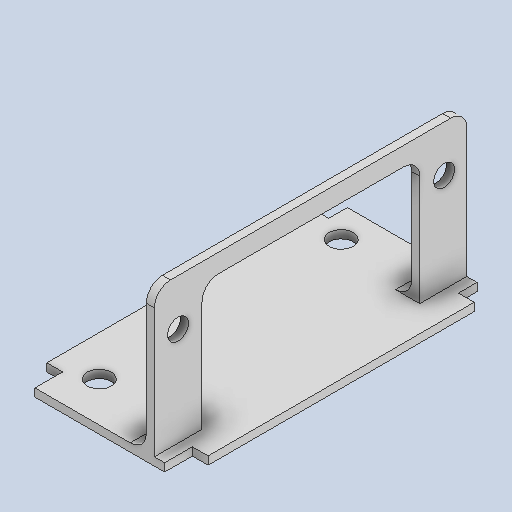
# Autodesk Inventor part: spekaer cover
Saved by Autodesk Inventor 2022.2 (Build 262287000, 287)
## iProperties
Created: 2022-02-22
Part Number: spekaer cover
Material: Generic
Document SubType Name: Modeling
Designer: ONG
Density: 1 g/cm^3
Appearance: Default
Author: ONG
Autodesk Inventor part; units mm, degrees
ref_plane "YZ Plane" through (0, 0, 0) normal (1, 0, 0) x (0, 1, 0)
ref_plane "XZ Plane" through (0, 0, 0) normal (0, 1, 0) x (-1, 0, 0)
ref_plane "XY Plane" through (0, 0, 0) normal (0, 0, 1) x (1, 0, 0)
sketch "Sketch1" plane through (0, 0, 0) normal (0, 1, 0) x (-1, 0, 0)
  line L0 (-10, -16.5) -> (10, -16.5)
  line L1 (10, -16.5) -> (10, 16.5)
  line L2 (10, 16.5) -> (-10, 16.5)
  line L3 (-10, 16.5) -> (-10, -16.5)
  line L4 (-10, -16.5) -> (10, 16.5) construction
  line L5 (10, -16.5) -> (-10, 16.5) construction
  point P0 (0, 0)
  dimension "d0" = 20
  dimension "d1" = 33
  constraints: 12 end point, 2 midpoint, 2 parallel, 1 horizontal, 1 perpendicular
  measures "d0" distance of L2.end L1.end
  measures "d1" distance of L1.end L0.end
extrude "Extrusion1" add sketch "Sketch1" along normal blind 1
sketch "Sketch2" plane through (0, 1, 0) normal (0, 1, 0) x (1, 0, 0)
  line L0 (0, 0) -> (0, 15)
  line L1 (0, 0) -> (0, -16.9855)
  line L2 (-8.0399, 11.188) -> (8.0399, 11.188)
  line L3 (8.0399, 11.188) -> (8.0399, 18.812)
  line L4 (8.0399, 18.812) -> (-8.0399, 18.812)
  line L5 (-8.0399, 18.812) -> (-8.0399, 11.188)
  line L6 (-8.0399, 11.188) -> (8.0399, 18.812) construction
  line L7 (8.0399, 11.188) -> (-8.0399, 18.812) construction
  line L8 (-8.0399, -19.9319) -> (8.0399, -19.9319)
  line L9 (8.0399, -19.9319) -> (8.0399, -14.0391)
  line L10 (8.0399, -14.0391) -> (-8.0399, -14.0391)
  line L11 (-8.0399, -14.0391) -> (-8.0399, -19.9319)
  line L12 (-8.0399, -19.9319) -> (8.0399, -14.0391) construction
  line L13 (8.0399, -19.9319) -> (-8.0399, -14.0391) construction
  dimension "d4" = 15
  constraints: 28 end point, 4 midpoint, 4 parallel, 2 horizontal, 2 perpendicular, 2 vertical, 1 point on line
  measures "d4" distance of L0.start L0.end
extrude "Extrusion2" add sketch "Sketch2" against normal blind 1
sketch "Sketch3" plane through (0, 1, 0) normal (0, 1, 0) x (1, 0, 0)
  line L0 (-8.0399, 18.812) -> (8.0399, 18.812) projected
  line L1 (6.7702, 18.812) -> (5.7702, 18.812)
  line L2 (5.7702, 18.812) -> (5.7702, 12.9733)
  line L3 (5.7702, 12.9733) -> (6.7702, 12.9733)
  line L4 (6.7702, 12.9733) -> (6.7702, 18.812)
  line L5 (8.0399, -19.9319) -> (-8.0399, -19.9319) projected
  line L6 (6.7702, -14.028) -> (5.7702, -14.028)
  line L7 (5.7702, -14.028) -> (5.7702, -19.9319)
  line L8 (5.7702, -19.9319) -> (6.7702, -19.9319)
  line L9 (6.7702, -19.9319) -> (6.7702, -14.028)
  point P0 (0, 0)
  dimension "d7" = 1
  constraints: 16 end point, 4 parallel, 2 horizontal, 2 perpendicular, 2 point on line
  measures "d7" distance of L3.end L2.end
extrude "Extrusion3" add sketch "Sketch3" along normal blind 18
fillet "Fillet1" radius 2 2 edges at (5.7702, 1, -15.8927) (5.7702, 1, 16.9799)
sketch "Sketch4" plane through (6.7702, 1, -12.9733) normal (1, 0, 0) x (0, 0, -1)
  circle A0 centre (2.9948, 12.1931) radius 1.1455
  circle A1 centre (-29.9076, 12.1931) radius 1.1628
  point P0 (-12.9733, -1)
  constraints: 2 centre point
extrude "Extrusion4" cut sketch "Sketch4" against normal blind 15
sketch "Sketch5" plane through (6.7702, 19, 14.028) normal (0, 0, -1) x (-1, 0, 0)
  line L0 (1, -16) -> (1, 0) projected
  line L1 (0, 0) -> (1, 0)
  line L2 (1, 0) -> (1, -2.3095)
  line L3 (1, -2.3095) -> (0, -2.3095)
  line L4 (0, -2.3095) -> (0, 0)
  point P0 (6.7702, -19)
  constraints: 8 end point, 2 parallel, 1 horizontal, 1 perpendicular, 1 point on line
extrude "Extrusion5" add sketch "Sketch5" along normal blind 30
fillet "Fillet2" radius 2 4 edges at (6.2702, 19, -18.812) (6.2702, 19, 19.9319) (6.2702, 16.6905, 14.028) (6.2702, 16.6905, -12.9733)
sketch "Sketch7" plane through (0, 1, 0) normal (0, 1, 0) x (1, 0, 0)
  line L0 (0, 0) -> (-5.0872, 0)
  line L1 (0, 0) -> (-5, 0)
  line L2 (-5, 0) -> (-5, -15)
  line L3 (-5, -15) -> (-5, 15)
  circle A0 centre (-5, 15) radius 1.5
  circle A1 centre (-5, -15) radius 1.5
  dimension "d19" = 5
  dimension "d20" = 15
  dimension "d21" = 30
  dimension "d22" = 3
  dimension "d23" = 3
  constraints: 8 end point, 2 centre point, 2 coincident, 2 point on line, 1 horizontal, 1 perpendicular
  measures "d19" distance of L0.start L1.end
  measures "d20" distance of L1.end L2.end
  measures "d21" distance of L2.end L3.end
  measures "d22" diameter of A0
  measures "d23" diameter of A1
extrude "Extrusion6" cut sketch "Sketch7" against normal through all
thread "Thread1" size "M2.5x0.45" class "6H" standard "ANSI Metric M Profile" full length
thread "Thread2" size "M2.3x0.45" class "6H" standard "ANSI Metric M Profile" full length
sketch "Sketch10" plane through (5.7702, 3, 14.028) normal (-1, 0, 0) x (0, 0, 1)
  point P0 (2.972, 10.25)
  point P1 (-30.028, 10.25)
hole "Hole3" at (5.7702, 13.25, 17) at (5.7702, 13.25, -16) direction (1, 0, 0) diameter 2.6 end through all
body "Solid1"
